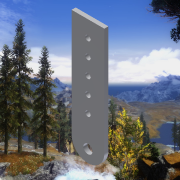
# Autodesk Inventor part: C18_TK_ClimberingSupportGusset
Saved by Autodesk Inventor 2015 SP1 (Build 190203100, 203)
## iProperties
Created: 2015-01-17
Part Number: C18_TK_ClimberingSupportGusset
Material: Aluminum 6061
Document SubType Name: Modeling
Designer: Administrator
Density: 2.71 g/cm^3
Appearance: Aluminum - Flat
Mass: 19.7578 g
Surface Area: 55.6812 cm^2
Volume: 7.29071 cm^3
Author: Administrator
Autodesk Inventor part; units mm, degrees
ref_plane "YZ Plane" through (0, 0, 0) normal (1, 0, 0) x (0, 1, 0)
ref_plane "XZ Plane" through (0, 0, 0) normal (0, 1, 0) x (-1, 0, 0)
ref_plane "XY Plane" through (0, 0, 0) normal (0, 0, 1) x (1, 0, 0)
sketch "Sketch1" plane through (0, 0, 0) normal (0, 0, 1) x (1, 0, 0)
  circle A0 centre (0, 0) radius 3.5687
  line L0 (-12.7, 61.849) -> (12.7, 61.849)
  line L1 (12.7, 61.849) -> (12.7, -9.525)
  line L2 (12.7, -9.525) -> (-12.7, -9.525)
  line L3 (-12.7, -9.525) -> (-12.7, 61.849)
  dimension "d0" = 7.1374
  dimension "d1" = 12.7
  dimension "d2" = 25.4
  dimension "d3" = 9.525
  dimension "d4" = 71.374
  constraints: 8 end point, 2 parallel, 1 centre point, 1 coincident, 1 horizontal, 1 perpendicular
  measures "d0" diameter of A0
  measures "d1" distance from line of point (0, 0) L3
  measures "d2" distance of L1.end L2.end
  measures "d3" distance from line of L2 point (0, 0)
  measures "d4" distance of L0.end L1.end
extrude "Extrusion1" add sketch "Sketch1" along normal mid plane 3.175
sketch "Sketch2" plane through (0, 0, 1.5875) normal (0, 0, 1) x (1, 0, 0)
  line L0 (-12.7, -9.525) -> (12.7, -9.525) projected
  point P0 (0, 46.609)
  point P1 (0, 33.909)
  point P2 (0, 59.309)
  point P3 (0, 72.009)
  dimension "d8" = 12.7
  dimension "d20" = 12.7
  dimension "d30" = 12.7
  dimension "d31" = 43.434
  measures "d8" distance of point (0, 33.909) point (0, 46.609)
  measures "d20" distance of point (0, 72.009) point (0, 59.309)
  measures "d30" distance of point (0, 59.309) point (0, 46.609)
  measures "d31" distance from line of L0 point (0, 33.909)
hole "Hole1" at (0, 46.609, 1.5875) at (0, 33.909, 1.5875) direction (0, 0, -1) diameter 4.0894 end through all
fillet "Fillet2" radius 12.7 2 edges at (12.7, -9.525, 0) (-12.7, -9.525, 0)
sketch "Sketch3" plane through (-12.7, 61.849, 1.5875) normal (0, 1, 0) x (1, 0, 0)
  line L0 (0, 3.175) -> (0, 0) projected
  line L1 (25.4, 0) -> (0, 0) projected
  line L2 (25.4, 0) -> (25.4, 3.175) projected
  line L3 (0, 3.175) -> (25.4, 3.175) projected
  point P0 (12.7, 1.5875)
extrude "Extrusion2" add sketch "Sketch3" along normal blind 25.4
hole "Hole2" at (0, 59.309, 1.5875) at (0, 72.009, 1.5875) direction (0, 0, -1) diameter 4.0894 end through all
body "Solid1"
